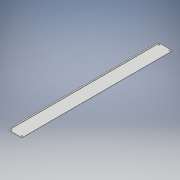
# Autodesk Inventor part: sideplate part 2
Saved by Autodesk Inventor 2018 (Build 220112000, 112)
## iProperties
Created: 2018-06-15
Part Number: sideplate part 2
Material: Generic
Document SubType Name: Sheet Metal
Designer: John Viljoen
Density: 1 g/cm^3
Sheet Metal Rule: Default_mm
Appearance: Default
Author: John Viljoen
Autodesk Inventor part; units mm, degrees
ref_plane "YZ Plane" through (0, 0, 0) normal (1, 0, 0) x (0, 1, 0)
ref_plane "XZ Plane" through (0, 0, 0) normal (0, 1, 0) x (-1, 0, 0)
ref_plane "XY Plane" through (0, 0, 0) normal (0, 0, 1) x (1, 0, 0)
sketch "Sketch1" plane through (0, 0, 0) normal (0, 0, 1) x (1, 0, 0)
  line L0 (0, 0) -> (29.621, 0)
  line L1 (29.621, 0) -> (29.621, 338.525)
  line L2 (29.621, 338.525) -> (0, 338.525)
  line L3 (0, 338.525) -> (0, 0)
  dimension "d0" = 29.621
  dimension "d1" = 338.525
  measures "d0" distance of L2.end L1.end
  measures "d1" distance of L1.end L0.end
extrude "Plate1" add sketch "Sketch1" along normal blind 0.5
sketch "Sketch2" plane through (-0.5764, 0, 0.6152) normal (-0.3842953, 0, -0.9232102) x (0, -1, 0)
  line L0 (-338.525, 0) -> (0, 0)
  line L1 (0, 0) -> (0, 2.0004)
  line L2 (0, 2.0004) -> (-338.525, 2.0004)
  line L3 (-338.525, 2.0004) -> (-338.525, 0)
  constraints: 6 end point, 1 horizontal, 1 perpendicular, 1 vertical
edge flange "Flange1" height 2.4 angle 22.6 thickness 0.5 bend radius 1.5 thickness toward (-0.3842953, 0, -0.9232102) relief tear relief width 0.5 relief depth 0.25 edges at (0, 169.2625, 0.5) wall of the first edge with corners at (-0.5764, 338.525, 0.6152) (-0.5764, 0, 0.6152) (-2.4232, 0, 1.3839) (-2.4232, 338.525, 1.3839)
bend "Bend1"
corner "Corner1"
sketch "Sketch3" plane through (29.621, 0, 0) normal (1, 0, 0) x (0, 0, -1)
  line L0 (0, 0) -> (-3.9531, 0)
  line L1 (-3.9531, 0) -> (-3.9531, 6.35)
  line L2 (-3.9531, 6.35) -> (0, 6.35)
  line L3 (0, 6.35) -> (0, 0)
  dimension "d13" = 6.35
  constraints: 8 end point, 2 parallel, 1 horizontal, 1 perpendicular
  measures "d13" distance of L0.end L1.end
extrude "Extrusion1" cut sketch "Sketch3" against normal through all
sketch "Sketch4" plane through (0, 0, 0.5) normal (0, 0, 1) x (1, 0, 0)
  line L0 (0, 6.35) -> (29.621, 6.35)
  line L1 (29.621, 6.35) -> (29.621, 0)
  line L2 (29.621, 0) -> (0, 0)
  line L3 (0, 0) -> (0, 6.35)
  constraints: 8 end point, 2 parallel, 1 horizontal, 1 perpendicular
extrude "Extrusion2" add sketch "Sketch4" against normal up to surface (0.5 mm away)
sketch "Sketch5" plane through (0, 0, 0.5) normal (0, 0, 1) x (1, 0, 0)
  line L0 (29.621, 0) -> (29.621, 338.525) projected
  line L1 (0, 6.35) -> (0, 338.525) projected
  line L2 (0, 0) -> (29.621, 0) projected
  line L3 (0, 0) -> (3.175, 0) construction
  line L4 (3.175, 0) -> (3.175, 3.175) construction
  line L5 (29.621, 0) -> (26.446, 0) construction
  line L6 (26.446, 0) -> (26.446, 3.175) construction
  line L7 (0, 338.525) -> (0, 335.35) construction
  line L8 (0, 335.35) -> (3.175, 335.35) construction
  line L9 (29.621, 338.525) -> (29.621, 335.35) construction
  line L10 (29.621, 335.35) -> (26.446, 335.35) construction
  circle A0 centre (3.175, 335.35) radius 1.25
  circle A1 centre (26.446, 335.35) radius 1.25
  line L11 (3.175, 3.175) -> (3.175, 3.35) construction
  line L12 (26.446, 3.175) -> (26.446, 3.35) construction
  circle A2 centre (26.446, 3.35) radius 1.25
  circle A3 centre (3.175, 3.35) radius 1.25
  dimension "d18" = 3.175
  dimension "d19" = 3.175
  dimension "d20" = 3.175
  dimension "d21" = 3.175
  dimension "d24" = 3.175
  dimension "d25" = 3.175
  dimension "d26" = 3.175
  dimension "d27" = 3.175
  dimension "d28" = 2.5
  dimension "d29" = 2.5
  dimension "d38" = 0.175
  dimension "d39" = 0.175
  dimension "d40" = 2.5
  dimension "d41" = 2.5
  constraints: 20 end point, 6 coincident, 4 centre point, 4 perpendicular, 4 point on line, 2 vertical
  measures "d18" distance of L2.start L3.end
  measures "d19" distance of L3.end L4.end
  measures "d20" distance of L0.start L5.end
  measures "d21" distance of L5.end L6.end
  measures "d24" distance of L1.end L7.end
  measures "d25" distance of L7.end L8.end
  measures "d26" distance of L0.end L9.end
  measures "d27" distance of L9.end L10.end
  measures "d28" diameter of A0
  measures "d29" diameter of A1
  measures "d38" distance of L11.start L11.end
  measures "d39" distance of L12.start L12.end
  measures "d40" diameter of A2
  measures "d41" diameter of A3
extrude "Extrusion3" cut sketch "Sketch5" against normal blind 10
sketch "Sketch6" plane through (0, 0, 0.5) normal (0, 0, 1) x (1, 0, 0)
  line L0 (0, 0) -> (35.9429, 0)
  line L1 (35.9429, 0) -> (35.9429, 0.175)
  line L2 (35.9429, 0.175) -> (0, 0.175)
  line L3 (0, 0.175) -> (0, 0)
  line L4 (0, 6.35) -> (-5.8334, 6.35)
  line L5 (-5.8334, 6.35) -> (-5.8334, 6.525)
  line L6 (-5.8334, 6.525) -> (0, 6.525)
  line L7 (0, 6.525) -> (0, 6.35)
  dimension "d32" = 0.175
  dimension "d33" = 0.175
  constraints: 16 end point, 4 parallel, 2 horizontal, 2 perpendicular
  measures "d32" distance of L1.end L0.end
  measures "d33" distance of L4.end L5.end
extrude "Extrusion4" cut sketch "Sketch6" against normal blind 10 and the other way blind 5
equation "\"d2\" = Thickness"
equation "\"d3\" = BendReliefWidth"
equation "\"d4\" = BendReliefDepth"
equation "\"d5\" = MinimumRemnant"
equation "\"d6\" = TransitionRadius"
equation "\"d10\" = CornerReliefSize"
equation "\"d11\" = GapSize"
equation "\"d12\" = JacobiRadiusSize"
equation "\"BendRadius\" = Thickness"
equation "\"BendReliefWidth\" = Thickness"
equation "\"BendReliefDepth\" = 0.5 * Thickness"
equation "\"CornerReliefSize\" = 4 * Thickness"
equation "\"MinimumRemnant\" = 2 * Thickness"
equation "\"TransitionRadius\" = BendRadius"
equation "\"JacobiRadiusSize\" = BendRadius"
equation "\"GapSize\" = Thickness"
equation "\"Thickness\" = 0.5"
body "Solid1"
